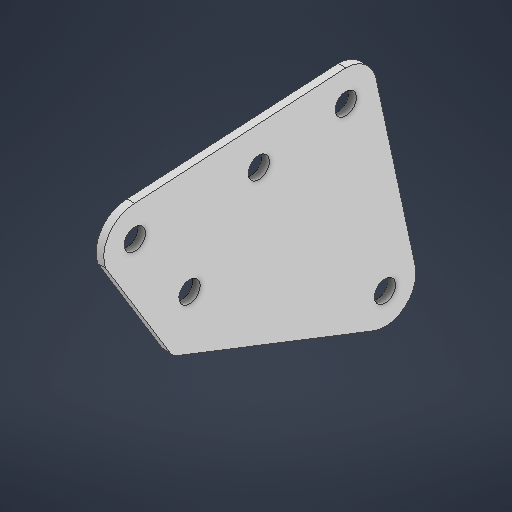
# Autodesk Inventor part: lbsupport
Saved by Autodesk Inventor 2025.2 (Build 292293000, 293)
## iProperties
Created: 2025-03-30
Part Number: lbsupport
Material: Generic
Document SubType Name: Modeling
Designer: roejo
Density: 1 g/cm^3
Appearance: Default
Author: roejo
Autodesk Inventor part; units mm, degrees
ref_plane "YZ Plane" through (0, 0, 0) normal (1, 0, 0) x (0, 1, 0)
ref_plane "XZ Plane" through (0, 0, 0) normal (0, 1, 0) x (-1, 0, 0)
ref_plane "XY Plane" through (0, 0, 0) normal (0, 0, 1) x (1, 0, 0)
sketch "Sketch1" plane through (0, 0, 0) normal (1, 0, 0) x (0, 1, 0)
  circle A0 centre (1.8217, 14.5615) radius 2.1844
  circle A1 centre (16.7653, 25.7818) radius 2.1844
  circle A2 centre (16.7653, 0.3818) radius 2.1844
  circle A3 centre (19.1795, -17.4456) radius 2.1844
  circle A4 centre (-18.0648, -25.4753) radius 2.1844
  circle A5 centre (19.1795, -17.4456) radius 6.35
  circle A6 centre (16.7653, 25.7818) radius 6.35
  circle A7 centre (-18.0648, -25.4753) radius 6.35
  line L0 (20.6395, -23.6254) -> (-16.7263, -31.6826)
  line L1 (25.5295, -17.4456) -> (23.1153, 25.7818)
  line L2 (14.5809, 31.7443) -> (-6.9779, 18.5698)
  line L3 (-8.2796, 17.0161) -> (-23.9793, -23.1643)
  arc A8 (-6.9779, 18.5698) -> (-8.2796, 17.0161) centre (-5.3223, 15.8607) ccw
  point P0 (0, 0)
  dimension "d0" = 12.7
  dimension "d1" = 12.7
  dimension "d2" = 12.7
  dimension "d3" = 3.175
  constraints: 9 centre point, 8 end point, 8 point on circle, 4 tangent, 3 coincident
  measures "d0" diameter of A5
  measures "d1" diameter of A6
  measures "d2" diameter of A7
  measures "d3" radius of A8
extrude "Extrusion1" add sketch "Sketch1" along normal blind 1.5875 contours A5 L1 | L0 A7 L3 A8 L2 A6 L1 A5 | A7 | A6 L2 picked at (18.545, -22.3352) picked at (14.1871, 29.9232)
body "Solid1"
